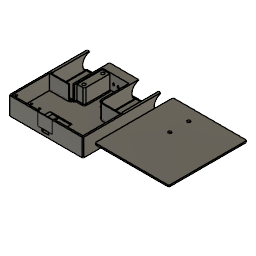
NeoLabs-Rocket-LaunchSystem (Autodesk Fusion 360 design; units mm, degrees)
part number: 2026-06-22-15-23-40-564
Autodesk Fusion 360 part; units mm, degrees
sketch "Sketch1" plane through (0, 0, 0) normal (0, 0, 1) x (1, 0, 0)
  line L0 (-60, -35) -> (39, -35)
  line L1 (39, -35) -> (39, 69.6198)
  line L2 (39, 69.6198) -> (-60, 69.6198)
  line L3 (-60, 69.6198) -> (-60, -35)
  circle A0 centre (-54.5, -30.5) radius 1.35
  circle A1 centre (-34.5, -30.5) radius 1.35
  circle A2 centre (-23.5, -30.5) radius 1.35
  circle A3 centre (-0.5, -30.5) radius 1.35
  dimension "d1" = 99
  dimension "d9" = 2.7
  dimension "d10" = 2.7
  dimension "d11" = 2.7
  dimension "d12" = 2.7
  constraint horizontal L0
  constraint vertical L1
  constraint horizontal L2
  constraint vertical L3
  measures "d1" distance of L0.start L0.end
  measures "d9" diameter of A0
  measures "d10" diameter of A1
  measures "d11" diameter of A2
  measures "d12" diameter of A3
extrude "Extrude1" add sketch "Sketch1" against normal blind 4 makes body 1
extrude "Extrude2" add sketch "Sketch1" along normal blind 6 and the other way blind 4 contours A0 | A1 | A2 | A3 bodies 1
sketch "Sketch2" plane through (0, 0, 0) normal (0, 0, 1) x (-1, 0, 0)
  line L0 (60, -69.6198) -> (60, 35)
  line L1 (60, 35) -> (-39, 35)
  line L2 (-39, 35) -> (-39, -69.6198)
  line L3 (-39, -69.6198) -> (60, -69.6198)
  circle A0 centre (0.5, 30.5) radius 1.35
  circle A1 centre (34.5, 30.5) radius 1.35
  circle A2 centre (54.5, 30.5) radius 1.35
  circle A3 centre (23.5, 30.5) radius 1.35
  line L4 (30.3925, -68.4602) -> (56.3925, -68.4602)
  line L5 (56.3925, -68.4602) -> (56.3925, -20.4602)
  line L6 (56.3925, -20.4602) -> (30.3925, -20.4602)
  line L7 (30.3925, -20.4602) -> (30.3925, -68.4602)
  line L8 (31.8289, -17.2317) -> (57.8727, -17.2317)
  line L9 (57.8727, -17.2317) -> (57.8727, -18.2915)
  line L10 (57.8727, -18.2915) -> (31.8289, -18.2915)
  line L11 (31.8289, -18.2915) -> (31.8289, -17.2317)
  line L12 (57.8615, -18.2915) -> (57.8615, -20.4602)
  line L13 (31.8289, -20.7915) -> (31.8289, -21.7915)
  line L14 (59.9993, -21.7915) -> (59.9993, -16.2915)
  line L15 (57.8615, -17.2317) -> (57.8615, -20.4602)
  line L16 (60, -69.6198) -> (58, -69.6198)
  line L17 (60, -21.7915) -> (60, -69.6198)
  line L18 (60, -21.7915) -> (59.9993, -21.7915)
  line L19 (57.9993, -16.2915) -> (57.9993, 33)
  line L20 (57.9993, 35) -> (59.9993, 35)
  line L21 (59.9993, 35) -> (59.9993, -16.2915)
  line L22 (-39, 35) -> (-37, 35)
  line L23 (-3, -69.6198) -> (-39, -69.6198)
  line L24 (-39, -69.6198) -> (-39, 35)
  line L25 (-3, -69.6198) -> (30.1003, -69.6198)
  line L26 (30.1003, -69.6198) -> (30.1003, -67.6198)
  line L27 (58, -69.6198) -> (56.8045, -69.6198)
  line L28 (56.8045, -69.6198) -> (56.8045, -67.6198)
  line L29 (30.3925, -20.4602) -> (57.8727, -20.4602)
  line L30 (57.8727, -20.4602) -> (57.8727, -18.2915)
  line L31 (57.8727, -18.2915) -> (30.3925, -18.2915)
  line L32 (30.3925, -18.2915) -> (30.3925, -20.4602)
  line L33 (-39, 35) -> (60, 35)
  line L34 (60, 35) -> (60, 33)
  line L35 (-39, 0.9412) -> (-39, 35)
  line L36 (60, 33) -> (59.9993, 33)
  line L37 (57.9993, 33) -> (-3, 33)
  line L38 (28.1003, -58.5213) -> (28.1003, -20.4602)
  line L39 (28.1003, -20.4602) -> (30.1003, -20.4602)
  line L40 (30.1003, -20.4602) -> (30.1003, -67.6198)
  line L41 (57.8727, -20.4602) -> (56.8045, -20.4602)
  line L42 (56.8045, -20.4602) -> (56.8045, -67.6198)
  line L43 (28.1003, -58.5213) -> (17.9963, -58.5213)
  line L44 (57.9993, -16.2915) -> (57.9993, -17.2317)
  line L45 (57.9993, -17.2317) -> (57.8727, -17.2317)
  line L46 (-9.1003, -20.4602) -> (-9.1003, -67.6198)
  line L47 (-9.1003, -69.6198) -> (-9.1003, -67.6198)
  line L48 (-35.8045, -20.4602) -> (-35.8045, -67.6198)
  line L49 (-35.8045, -69.6198) -> (-35.8045, -67.6198)
  line L50 (-36.8615, -17.2317) -> (-36.8615, -20.4602)
  line L51 (-35.3925, -20.4602) -> (-9.3925, -20.4602)
  line L52 (-36.8727, -20.4602) -> (-35.8045, -20.4602)
  line L53 (-9.3925, -20.4602) -> (-36.8727, -20.4602)
  line L54 (-36.8727, -18.2915) -> (-10.8289, -18.2915)
  line L55 (-10.8289, -17.2317) -> (-36.8727, -17.2317)
  line L56 (-36.8727, -18.2915) -> (-9.3925, -18.2915)
  line L57 (-9.3925, -18.2915) -> (-9.3925, -20.4602)
  line L58 (-10.8289, -18.2915) -> (-10.8289, -17.2317)
  line L59 (-7.1003, -20.4602) -> (-9.1003, -20.4602)
  line L60 (-7.1003, -58.5213) -> (-7.1003, -20.4602)
  line L61 (-39, -21.7915) -> (-39, -69.6198)
  line L62 (-39, -69.6198) -> (-37, -69.6198)
  line L63 (-37, -69.6198) -> (-35.8045, -69.6198)
  line L64 (-39, -21.7915) -> (-39, 35)
  line L65 (-37, 35) -> (10.5, 35)
  line L66 (-3, 33) -> (-36.8727, 33)
  line L67 (-36.8727, -17.2317) -> (-36.8727, 33)
  line L68 (-7.1003, -58.5213) -> (3.0037, -58.5213)
  line L69 (3.0037, -58.5213) -> (17.9963, -58.5213)
  dimension "d27" = 26
  dimension "d28" = 48
  dimension "d34" = 2
  dimension "d35" = 2
  dimension "d36" = 2
  constraint horizontal L4
  constraint vertical L5
  constraint horizontal L6
  constraint vertical L7
  constraint horizontal L8
  constraint vertical L9
  constraint horizontal L10
  constraint vertical L11
  constraint coincident L10 L12.start
  constraint perpendicular L10 L12
  constraint vertical L13
  constraint vertical L14
  constraint vertical L15
  constraint horizontal L16
  constraint vertical L17
  constraint coincident L0.start L3.end
  constraint vertical L19
  constraint horizontal L20
  constraint vertical L21
  constraint horizontal L22
  constraint horizontal L23
  constraint vertical L24
  constraint coincident L1.end L2.start
  constraint horizontal L25
  constraint vertical L26
  constraint horizontal L27
  constraint vertical L28
  constraint horizontal L29
  constraint vertical L30
  constraint horizontal L31
  constraint vertical L32
  constraint horizontal L33
  constraint vertical L34
  constraint horizontal L36
  constraint vertical L35
  constraint coincident L0 L34.end
  constraint coincident L21 L36.end
  constraint collinear L36 L37
  constraint vertical L38
  constraint horizontal L39
  constraint vertical L40
  constraint horizontal L41
  constraint vertical L42
  constraint coincident L29 L12.end
  constraint horizontal L43
  constraint perpendicular L8 L44
  constraint perpendicular L15 L45
  constraint coincident L8 L15.start
  constraint midpoint L33 L65.end
  constraint perpendicular L66 L67
  measures "d27" distance of L4.start L4.end
  measures "d28" distance of L4.start L6.end
  measures "d34" distance of L0.start L16.end
  measures "d35" distance of L14.end L19.start
  measures "d36" distance of L1.end L22.end
extrude "Extrude3" add sketch "Sketch2" along normal blind 10 contours L8 L10 L11 L15 L31 | L50 L54 L55 L56 L58 bodies 1
extrude "Extrude5" add sketch "Sketch2" along normal blind 2 contours L6 L10 L12 L15 L29 L31 L32 L41 | L50 L51 L52 L53 L54 L56 L57 bodies 1
extrude "Extrude6" add sketch "Sketch2" along normal blind 20 contours L0 L1 L2 L3 L9 L14 L16 L17 L19 L20 L21 L22 L23 L24 L27 L28 L29 L30 L33 L34 L35 L37 L41 L42 L44 L45 L48 L49 L50 L52 L53 L55 L61 L62 L63 L64 L65 L66 L67 | L3 L23 L25 L26 L38 L39 L40 L43 L46 L47 L59 L60 L68 L69 | L10 L12 L15 L29 L30 L31 L41 | L8 L9 L10 L15 L31 | L8 L10 L11 L15 L31 | L50 L54 L55 L56 L58 | A0 | A1 | A2 | A3 bodies 1
sketch "Sketch4" plane through (-60, 0, 0) normal (-1, 0, 0) x (0, -1, 0)
  line L0 (-69.6198, 20) -> (-69.6198, -4)
  line L1 (-69.6198, -4) -> (35, -4)
  line L2 (35, -4) -> (35, 0)
  line L3 (35, 0) -> (-21.7915, 0)
  line L4 (-21.7915, 0) -> (-21.7915, 20)
  line L5 (-21.7915, 20) -> (-69.6198, 20)
  circle A0 centre (-72, 8) radius 10.4908
extrude "Extrude8" cut sketch "Sketch4" against normal blind 106 contours L0 A0 | L0 A0 bodies 1
sketch "Sketch10" plane through (0, 58.5213, 0) normal (0, -1, 0) x (1, 0, 0)
  line L0 (-28.1003, 0) -> (7.1003, 0)
  line L1 (7.1003, 0) -> (7.1003, 20)
  line L2 (7.1003, 20) -> (-28.1003, 20)
  line L3 (-28.1003, 20) -> (-28.1003, 0)
  line L4 (9, 8.3056) -> (-30, 8.3056)
  line L5 (-10.5, 8.3056) -> (-10.5, 11)
  line L6 (-6.2556, 8.3056) -> (-7.4122, 10.4298)
  line L7 (-7.5876, 10.4301) -> (-8.7556, 8.3056)
  arc A0 (-8.7556, 8.3056) -> (-6.2556, 8.3056) centre (-7.5056, 8.3056) ccw
  arc A1 (-7.4122, 10.4298) -> (-7.5876, 10.4301) centre (-7.5, 10.382) ccw
  line L8 (-13.4124, 10.4301) -> (-12.2444, 8.3056)
  line L9 (-14.7444, 8.3056) -> (-13.5878, 10.4298)
  arc A2 (-13.4124, 10.4301) -> (-13.5878, 10.4298) centre (-13.5, 10.382) ccw
  arc A3 (-14.7444, 8.3056) -> (-12.2444, 8.3056) centre (-13.4944, 8.3056) ccw
  dimension "d92" = 2.5
  dimension "d93" = 0.1
  constraint perpendicular L3 L4
  constraint midpoint L4 L5.start
  constraint perpendicular L4 L5
  constraint coincident L4 A0.centre
  constraint coincident L4 L6.start
  constraint coincident L4 L7.end
  constraint tangent L6 A1
  constraint tangent L7 A1
  constraint symmetric L5 L6.start L9.start
  constraint symmetric L5 L7.end L8.end
  constraint symmetric L5 A0 A3
  constraint symmetric L5 L6.end L9.end
  constraint symmetric L5 L7.start L8.start
  constraint symmetric L5 A1 A2
  measures "d92" diameter of A0
  measures "d93" radius of A1
extrude "Extrude15" cut sketch "Sketch10" against normal blind 10 contours L4 L8 L9 A2 | L4 A3 | L4 A0 | L4 L6 L7 A1 bodies 1
fillet "Fillet2" radius 1 8 edges at (37.4022, 69.6198, 18.2172) (-10.5, 69.6198, 18.2172) (-58.4022, 69.6198, 18.2172) (-10.5, 69.6198, -2.2172) (-30.1003, 61.8033, 10.4663) (-56.8045, 61.8033, 10.4663) (35.8045, 61.8033, 10.4663) (9.1003, 61.8033, 10.4663) on bodies 1
sketch "Sketch5" plane through (0, 0, 0) normal (0, 0, 1) x (-1, 0, 0)
  line L0 (6.8, 32.85) -> (15.8, 32.85)
  line L1 (15.8, 32.85) -> (6.8, 32.85)
  line L2 (6.8, 32.85) -> (6.8, 37.441)
  line L3 (6.8, 37.441) -> (15.8, 37.441)
  line L4 (15.8, 37.441) -> (15.8, 32.85)
  circle A0 centre (54.5, 30.5) radius 1.35
  circle A1 centre (34.5, 30.5) radius 1.35
  circle A2 centre (0.5, 30.5) radius 1.35
  circle A3 centre (23.5, 30.5) radius 1.35
  line L5 (29.1003, -65.2135) -> (57.8045, -65.2135)
  spline S0 degree 3 poles (57.8045, -65.2135) (57.6964, -65.2135) (57.5714, -65.179) (57.3554, -65.0637) (57.235, -64.9522) (57.0463, -64.708) (56.9546, -64.5234) (56.8406, -64.1757) (56.8045, -63.9456) (56.8045, -63.7515) knots 0.358129 0.358129 0.358129 0.358129 0.39055 0.39055 0.431579 0.431579 0.483124 0.483124 0.541351 0.541351 0.541351 0.541351
  line L6 (56.8045, -63.7515) -> (56.8045, -20.4602)
  line L7 (56.8045, -20.4602) -> (30.3925, -20.4602)
  line L8 (30.3925, -20.4602) -> (30.3925, -18.2915)
  line L9 (30.3925, -18.2915) -> (31.8289, -18.2915)
  line L10 (31.8289, -18.2915) -> (31.8289, -17.2317)
  line L11 (31.8289, -17.2317) -> (57.9993, -17.2317)
  line L12 (57.9993, -17.2317) -> (57.9993, 33)
  line L13 (57.9993, 33) -> (-36.8727, 33)
  line L14 (-7.1003, -58.5213) -> (28.1003, -58.5213)
  line L15 (28.1003, -58.5213) -> (28.1003, -20.4602)
  line L16 (28.1003, -20.4602) -> (30.1003, -20.4602)
  line L17 (30.1003, -20.4602) -> (30.1003, -63.7515)
  spline S1 degree 3 poles (30.1003, -63.7515) (30.1003, -63.9456) (30.0641, -64.1757) (29.9501, -64.5234) (29.8585, -64.708) (29.6697, -64.9522) (29.5493, -65.0637) (29.3333, -65.179) (29.2083, -65.2135) (29.1003, -65.2135) knots 0.174906 0.174906 0.174906 0.174906 0.233133 0.233133 0.284679 0.284679 0.325708 0.325708 0.358129 0.358129 0.358129 0.358129
  line L18 (-36.8727, 33) -> (-36.8727, -17.2317)
  line L19 (-36.8727, -17.2317) -> (-10.8289, -17.2317)
  line L20 (-10.8289, -17.2317) -> (-10.8289, -18.2915)
  line L21 (-10.8289, -18.2915) -> (-9.3925, -18.2915)
  line L22 (-9.3925, -18.2915) -> (-9.3925, -20.4602)
  line L23 (-9.3925, -20.4602) -> (-35.8045, -20.4602)
  line L24 (-35.8045, -20.4602) -> (-35.8045, -63.7515)
  line L25 (-9.1003, -63.7515) -> (-9.1003, -20.4602)
  line L26 (-9.1003, -20.4602) -> (-7.1003, -20.4602)
  line L27 (-7.1003, -20.4602) -> (-7.1003, -58.5213)
  spline S2 degree 3 poles (-35.8045, -63.7515) (-35.8045, -63.9456) (-35.8406, -64.1757) (-35.9546, -64.5234) (-36.0463, -64.708) (-36.235, -64.9522) (-36.3554, -65.0637) (-36.5714, -65.179) (-36.6964, -65.2135) (-36.8045, -65.2135) knots 0.174906 0.174906 0.174906 0.174906 0.233133 0.233133 0.284679 0.284679 0.325708 0.325708 0.358129 0.358129 0.358129 0.358129
  line L28 (-36.8045, -65.2135) -> (-8.1003, -65.2135)
  spline S3 degree 3 poles (-8.1003, -65.2135) (-8.2083, -65.2135) (-8.3333, -65.179) (-8.5493, -65.0637) (-8.6697, -64.9522) (-8.8585, -64.708) (-8.9501, -64.5234) (-9.0641, -64.1757) (-9.1003, -63.9456) (-9.1003, -63.7515) knots 0.358129 0.358129 0.358129 0.358129 0.39055 0.39055 0.431579 0.431579 0.483124 0.483124 0.541351 0.541351 0.541351 0.541351
  dimension "d60" = 9
  constraint horizontal L1
  constraint vertical L2
  constraint horizontal L3
  constraint vertical L4
  measures "d60" distance of L0.start L0.end
extrude "Extrude9" cut sketch "Sketch5" along normal blind 3.2 contours L2 L3 L4 L13 bodies 1
sketch "Sketch6" plane through (0, 0, 20) normal (0, 0, 1) x (-1, 0, 0)
  line L0 (56.8045, -69.6198) -> (60, -69.6198)
  line L1 (60, -69.6198) -> (60, -21.7915)
  line L2 (60, -21.7915) -> (59.9993, -21.7915)
  line L3 (59.9993, -21.7915) -> (59.9993, 35)
  line L4 (59.9993, 35) -> (-39, 35)
  line L5 (-39, 35) -> (-39, -69.6198)
  line L6 (21.6224, 33) -> (2.3035, 33)
  line L7 (2.3035, 33) -> (2.3035, 34.4706)
  line L8 (2.3035, 34.4706) -> (21.6224, 34.4706)
  line L9 (21.6224, 34.4706) -> (21.6224, 33)
  line L10 (-36.8727, 33) -> (57.9993, 33)
  line L11 (57.9993, 33) -> (57.9993, -17.2317)
  line L12 (57.9993, -17.2317) -> (31.8289, -17.2317)
  line L13 (31.8289, -17.2317) -> (31.8289, -18.2915)
  line L14 (31.8289, -18.2915) -> (57.8615, -18.2915)
  line L15 (57.8615, -18.2915) -> (57.8615, -20.4602)
  line L16 (57.8615, -20.4602) -> (56.8045, -20.4602)
  line L17 (56.8045, -20.4602) -> (56.8045, -69.6198)
  line L18 (-39, -69.6198) -> (-35.8045, -69.6198)
  line L19 (-36.8615, -18.2915) -> (-10.8289, -18.2915)
  line L20 (-10.8289, -18.2915) -> (-10.8289, -17.2317)
  line L21 (-10.8289, -17.2317) -> (-36.8727, -17.2317)
  line L22 (-36.8727, -17.2317) -> (-36.8727, 33)
  line L23 (-35.8045, -69.6198) -> (-35.8045, -20.4602)
  line L24 (-35.8045, -20.4602) -> (-36.8615, -20.4602)
  line L25 (-36.8615, -20.4602) -> (-36.8615, -18.2915)
  constraint horizontal L6
  constraint vertical L7
  constraint horizontal L8
  constraint vertical L9
extrude "Extrude10" cut sketch "Sketch6" against normal blind 17 contours L6 L7 L8 L9 L10 bodies 1
fillet "Fillet3" radius 0.5 4 edges at (-1.7586, -30.0118, 0) (-24.7586, -30.0118, 0) (-35.7586, -30.0118, 0) (-55.7586, -30.0118, 0) on bodies 1
sketch "Sketch7" plane through (0, 0, 0) normal (0, 0, 1) x (-1, 0, 0)
  circle A0 centre (34.5, 30.5) radius 1.85
  circle A1 centre (0.5, 30.5) radius 1.85
  line L0 (29.1003, -65.2135) -> (57.8045, -65.2135)
  spline S0 degree 3 poles (57.8045, -65.2135) (57.6964, -65.2135) (57.5714, -65.179) (57.3554, -65.0637) (57.235, -64.9522) (57.0463, -64.708) (56.9546, -64.5234) (56.8406, -64.1757) (56.8045, -63.9456) (56.8045, -63.7515) knots 0.358129 0.358129 0.358129 0.358129 0.39055 0.39055 0.431579 0.431579 0.483124 0.483124 0.541351 0.541351 0.541351 0.541351
  line L1 (56.8045, -63.7515) -> (56.8045, -20.4602)
  line L2 (56.8045, -20.4602) -> (30.3925, -20.4602)
  line L3 (30.3925, -20.4602) -> (30.3925, -18.2915)
  line L4 (30.3925, -18.2915) -> (31.8289, -18.2915)
  line L5 (31.8289, -18.2915) -> (31.8289, -17.2317)
  line L6 (31.8289, -17.2317) -> (57.9993, -17.2317)
  line L7 (57.9993, -17.2317) -> (57.9993, 33)
  line L8 (57.9993, 33) -> (15.8, 33)
  line L9 (15.8, 33) -> (15.8, 35)
  line L10 (15.8, 35) -> (6.8, 35)
  line L11 (6.8, 35) -> (6.8, 33)
  line L12 (6.8, 33) -> (-36.8727, 33)
  line L13 (-7.1003, -58.5213) -> (28.1003, -58.5213)
  line L14 (28.1003, -58.5213) -> (28.1003, -20.4602)
  line L15 (28.1003, -20.4602) -> (30.1003, -20.4602)
  line L16 (30.1003, -20.4602) -> (30.1003, -63.7515)
  spline S1 degree 3 poles (30.1003, -63.7515) (30.1003, -63.9456) (30.0641, -64.1757) (29.9501, -64.5234) (29.8585, -64.708) (29.6697, -64.9522) (29.5493, -65.0637) (29.3333, -65.179) (29.2083, -65.2135) (29.1003, -65.2135) knots 0.174906 0.174906 0.174906 0.174906 0.233133 0.233133 0.284679 0.284679 0.325708 0.325708 0.358129 0.358129 0.358129 0.358129
  circle A2 centre (23.5, 30.5) radius 1.85
  circle A3 centre (54.5, 30.5) radius 1.85
  circle A4 centre (22.12, -52.8277) radius 2.05
  line L17 (27, -57) -> (17, -57)
  line L18 (17, -57) -> (17, -23)
  line L19 (17, -23) -> (27, -23)
  line L20 (27, -23) -> (27, -57)
  circle A5 centre (22.0931, -27.4434) radius 2.05
  line L21 (-36.8727, 33) -> (-36.8727, -17.2317)
  line L22 (-36.8727, -17.2317) -> (-10.8289, -17.2317)
  line L23 (-10.8289, -17.2317) -> (-10.8289, -18.2915)
  line L24 (-10.8289, -18.2915) -> (-9.3925, -18.2915)
  line L25 (-9.3925, -18.2915) -> (-9.3925, -20.4602)
  line L26 (-9.3925, -20.4602) -> (-35.8045, -20.4602)
  line L27 (-35.8045, -20.4602) -> (-35.8045, -63.7515)
  line L28 (-9.1003, -63.7515) -> (-9.1003, -20.4602)
  line L29 (-9.1003, -20.4602) -> (-7.1003, -20.4602)
  line L30 (-7.1003, -20.4602) -> (-7.1003, -58.5213)
  spline S2 degree 3 poles (-35.8045, -63.7515) (-35.8045, -63.9456) (-35.8406, -64.1757) (-35.9546, -64.5234) (-36.0463, -64.708) (-36.235, -64.9522) (-36.3554, -65.0637) (-36.5714, -65.179) (-36.6964, -65.2135) (-36.8045, -65.2135) knots 0.174906 0.174906 0.174906 0.174906 0.233133 0.233133 0.284679 0.284679 0.325708 0.325708 0.358129 0.358129 0.358129 0.358129
  line L31 (-36.8045, -65.2135) -> (-8.1003, -65.2135)
  spline S3 degree 3 poles (-8.1003, -65.2135) (-8.2083, -65.2135) (-8.3333, -65.179) (-8.5493, -65.0637) (-8.6697, -64.9522) (-8.8585, -64.708) (-8.9501, -64.5234) (-9.0641, -64.1757) (-9.1003, -63.9456) (-9.1003, -63.7515) knots 0.358129 0.358129 0.358129 0.358129 0.39055 0.39055 0.431579 0.431579 0.483124 0.483124 0.541351 0.541351 0.541351 0.541351
  dimension "d67" = 4.1
  dimension "d70" = 4.1
  constraint horizontal L17
  constraint vertical L18
  constraint horizontal L19
  constraint vertical L20
  measures "d67" diameter of A4
  measures "d70" diameter of A5
extrude "Extrude11" add sketch "Sketch7" along normal blind 20 contours L17 L18 L19 L20 bodies 1
extrude "Extrude12" add sketch "Sketch7" along normal blind 14 contours A4 | A5 bodies 1
fillet "Fillet4" radius 2 1 edges at (-17, 23, 10) on bodies 1
fillet "Fillet5" radius 0.5 8 edges at (-30.1003, 20.4602, 10) (-31.8289, 18.2915, 11) (-31.8289, 17.2317, 10) (-28.1003, 20.4602, 10) (7.1003, 20.4602, 10) (9.1003, 20.4602, 10) (10.8289, 18.2915, 11) (10.8289, 17.2317, 10) on bodies 1
fillet "Fillet6" radius 0.25 2 edges at (-30.3925, 18.2915, 1) (9.3925, 18.2915, 1) on bodies 1
fillet "Fillet7" radius 1 3 edges at (-17, 41, 0) (-17.5858, 23.5858, 0) (-23, 23, 0) on bodies 1
fillet "Fillet8" radius 0.5 16 edges at (-57.0463, 64.6852, 0) (-56.8045, 42.1058, 0) (-28.1003, 39.7407, 0) (-28.2467, 20.6066, 0) (-29.1003, 20.4602, 0) (-29.9538, 20.6066, 0) (-30.1003, 42.3558, 0) (-29.8584, 64.6852, 0) (8.8584, 64.6852, 0) (9.1003, 42.3558, 0) (8.9538, 20.6066, 0) (8.1003, 20.4602, 0) (7.2467, 20.6066, 0) (7.1003, 39.7407, 0) (35.8045, 42.1058, 0) (36.0463, 64.6852, 0) on bodies 1
chamfer "Chamfer1" distance 1 angle 45 13 edges at (39, -35, 8) (39, 69.6198, -3.4912) (39, 69.4242, -2.3883) (39, 61.5092, 8) (39, 69.4242, 18.3883) (39, 69.6198, 19.4912) (-59.9993, -35, 10) (-60, -35, -2) (-60, 69.6198, 19.4912) (-60, 69.4242, 18.3883) (-60, 61.5092, 8) (-60, 69.4242, -2.3883) (-60, 69.6198, -3.4912) on bodies 1
sketch "Sketch9" plane through (0, 0, 0) normal (0, 0, 1) x (-1, 0, 0)
  line L0 (27, -22) -> (27, -57)
  line L1 (27, -57) -> (16, -57)
  line L2 (16, -57) -> (16, -25)
  arc A0 (19, -22) -> (16, -25) centre (19, -25) ccw
  line L3 (19, -22) -> (27, -22)
  circle A1 centre (54.5, 30.5) radius 1.85
  circle A2 centre (23.5, 30.5) radius 1.85
  line L4 (27.6003, -58.5213) -> (27.6003, -20.9602)
  arc A3 (28.6003, -19.9602) -> (27.6003, -20.9602) centre (28.6003, -20.9602) ccw
  line L5 (28.6003, -19.9602) -> (29.6003, -19.9602)
  arc A4 (30.3925, -20.3499) -> (29.6003, -19.9602) centre (29.6003, -20.9602) ccw
  line L6 (30.3925, -20.3499) -> (30.3925, -18.5415)
  arc A5 (30.6425, -18.2915) -> (30.3925, -18.5415) centre (30.6425, -18.5415) ccw
  line L7 (30.6425, -18.2915) -> (31.8289, -18.2915)
  line L8 (31.8289, -18.2915) -> (31.8289, -17.7317)
  arc A6 (32.3289, -17.2317) -> (31.8289, -17.7317) centre (32.3289, -17.7317) ccw
  line L9 (32.3289, -17.2317) -> (57.9993, -17.2317)
  line L10 (57.9993, -17.2317) -> (57.9993, 33)
  line L11 (57.9993, 33) -> (15.8, 33)
  line L12 (15.8, 33) -> (15.8, 35)
  line L13 (15.8, 35) -> (6.8, 35)
  line L14 (6.8, 35) -> (6.8, 33)
  line L15 (6.8, 33) -> (-36.8727, 33)
  line L16 (-6.6003, -58.5213) -> (27.6003, -58.5213)
  circle A7 centre (0.5, 30.5) radius 1.85
  circle A8 centre (34.5, 30.5) radius 1.85
  line L17 (10.6673, -61.4434) -> (10.6673, -26.1703) construction
  line L18 (10.6673, -26.1703) -> (0.8534, -26.1703) construction
  line L19 (0.8534, -26.1703) -> (0.8534, -61.4434) construction
  line L20 (0.8534, -61.4434) -> (10.6673, -61.4434) construction
  line L21 (-36.8727, 33) -> (-36.8727, -17.2317)
  line L22 (-36.8727, -17.2317) -> (-11.3289, -17.2317)
  line L23 (-10.8289, -17.7317) -> (-10.8289, -18.2915)
  line L24 (-10.8289, -18.2915) -> (-9.6425, -18.2915)
  line L25 (-9.3925, -18.5415) -> (-9.3925, -20.3499)
  arc A9 (-10.8289, -17.7317) -> (-11.3289, -17.2317) centre (-11.3289, -17.7317) ccw
  arc A10 (-9.3925, -18.5415) -> (-9.6425, -18.2915) centre (-9.6425, -18.5415) ccw
  line L26 (-6.6003, -20.9602) -> (-6.6003, -58.5213)
  arc A11 (-8.6003, -19.9602) -> (-9.3925, -20.3499) centre (-8.6003, -20.9602) ccw
  line L27 (-8.6003, -19.9602) -> (-7.6003, -19.9602)
  arc A12 (-6.6003, -20.9602) -> (-7.6003, -19.9602) centre (-7.6003, -20.9602) ccw
  dimension "d88" = 5
  text T0 "Made by Neo" font "Arial" height 5 align centre middle in box 35.273 x 9.8139 at (10.6673, -61.4434) x (0, 1) y (-1, 0) spacing 1 kerned
extrude "Extrude14" cut sketch "Sketch9" against normal blind 1 text T0 bodies 1
sketch "Sketch11" plane through (0, 0, 0) normal (0, 0, 1) x (-1, 0, 0)
  circle A0 centre (34.5, 30.5) radius 1.85
  circle A1 centre (0.5, 30.5) radius 1.85
  line L0 (27.6003, -58.5213) -> (27.6003, -20.9602)
  arc A2 (28.6003, -19.9602) -> (27.6003, -20.9602) centre (28.6003, -20.9602) ccw
  line L1 (28.6003, -19.9602) -> (29.6003, -19.9602)
  arc A3 (30.3925, -20.3499) -> (29.6003, -19.9602) centre (29.6003, -20.9602) ccw
  line L2 (30.3925, -20.3499) -> (30.3925, -18.5415)
  arc A4 (30.6425, -18.2915) -> (30.3925, -18.5415) centre (30.6425, -18.5415) ccw
  line L3 (30.6425, -18.2915) -> (31.8289, -18.2915)
  line L4 (31.8289, -18.2915) -> (31.8289, -17.7317)
  arc A5 (32.3289, -17.2317) -> (31.8289, -17.7317) centre (32.3289, -17.7317) ccw
  line L5 (32.3289, -17.2317) -> (57.9993, -17.2317)
  line L6 (57.9993, -17.2317) -> (57.9993, 33)
  line L7 (57.9993, 33) -> (15.8, 33)
  line L8 (15.8, 33) -> (15.8, 35)
  line L9 (15.8, 35) -> (6.8, 35)
  line L10 (6.8, 35) -> (6.8, 33)
  line L11 (6.8, 33) -> (-36.8727, 33)
  line L12 (-36.8727, 33) -> (-36.8727, -17.2317)
  line L13 (-36.8727, -17.2317) -> (-11.3289, -17.2317)
  line L14 (-10.8289, -17.7317) -> (-10.8289, -18.2915)
  line L15 (-10.8289, -18.2915) -> (-9.6425, -18.2915)
  line L16 (-9.3925, -18.5415) -> (-9.3925, -20.3499)
  line L17 (-6.6003, -58.5213) -> (27.6003, -58.5213)
  circle A6 centre (23.5, 30.5) radius 1.85
  circle A7 centre (54.5, 30.5) radius 1.85
  line L18 (27, -22) -> (27, -57)
  line L19 (27, -57) -> (16, -57)
  line L20 (16, -57) -> (16, -25)
  arc A8 (19, -22) -> (16, -25) centre (19, -25) ccw
  line L21 (19, -22) -> (27, -22)
  line L22 (0.1021, -56.2744) -> (4.3585, -56.2744)
  line L23 (4.3585, -56.2744) -> (4.3585, -56.9122)
  line L24 (4.3585, -56.9122) -> (-0.6415, -56.9122)
  line L25 (-0.6415, -56.9122) -> (-0.6415, -55.9163)
  line L26 (-0.6415, -55.9163) -> (2.8988, -54.7328)
  spline S0 degree 3 poles (2.8988, -54.7328) (3.0427, -54.6852) (3.2889, -54.6038) (3.5362, -54.5263) (3.6389, -54.4941) knots 0 0 0 0 0.045488 0.077767 0.077767 0.077767 0.077767
  spline S1 degree 3 poles (3.6389, -54.4941) (3.5265, -54.458) (3.2585, -54.3719) (2.9921, -54.2809) (2.8374, -54.2281) knots 0 0 0 0 0.035404 0.084451 0.084451 0.084451 0.084451
  line L27 (2.8374, -54.2281) -> (-0.6415, -53.0309)
  line L28 (-0.6415, -53.0309) -> (-0.6415, -52.1408)
  line L29 (-0.6415, -52.1408) -> (4.3585, -52.1408)
  line L30 (4.3585, -52.1408) -> (4.3585, -52.7785)
  line L31 (4.3585, -52.7785) -> (0.1737, -52.7785)
  line L32 (0.1737, -52.7785) -> (4.3585, -54.2315)
  line L33 (4.3585, -54.2315) -> (4.3585, -54.8283)
  line L34 (4.3585, -54.8283) -> (0.1021, -56.2744)
  line L35 (-0.6415, -44.3474) -> (4.3585, -44.3474)
  line L36 (4.3585, -44.3474) -> (4.3585, -44.917)
  line L37 (4.3585, -44.917) -> (3.9015, -44.917)
  spline S2 degree 3 poles (3.9015, -44.917) (4.0587, -45.0468) (4.3773, -45.3099) (4.4192, -45.7214) (4.4404, -45.93) knots 0 0 0 0 0.058684 0.118957 0.118957 0.118957 0.118957
  spline S3 degree 3 poles (4.4404, -45.93) (4.4304, -46.0715) (4.4104, -46.3548) (4.2713, -46.6024) (4.2017, -46.7264) knots 0 0 0 0 0.041993 0.084065 0.084065 0.084065 0.084065
  spline S4 degree 3 poles (4.2017, -46.7264) (4.1127, -46.8413) (3.9307, -47.0764) (3.6687, -47.2172) (3.5349, -47.2891) knots 0 0 0 0 0.043095 0.088123 0.088123 0.088123 0.088123
  spline S5 degree 3 poles (3.5349, -47.2891) (3.3833, -47.3473) (3.0667, -47.4687) (2.7276, -47.4818) (2.5509, -47.4886) knots 0 0 0 0 0.048374 0.101007 0.101007 0.101007 0.101007
  spline S6 degree 3 poles (2.5509, -47.4886) (2.3769, -47.4821) (2.04, -47.4696) (1.7211, -47.3606) (1.5669, -47.3079) knots 0 0 0 0 0.051911 0.100523 0.100523 0.100523 0.100523
  spline S7 degree 3 poles (1.5669, -47.3079) (1.4294, -47.2418) (1.1617, -47.1131) (0.9789, -46.8793) (0.8899, -46.7656) knots 0 0 0 0 0.045081 0.087788 0.087788 0.087788 0.087788
  spline S8 degree 3 poles (0.8899, -46.7656) (0.8213, -46.6408) (0.6827, -46.389) (0.664, -46.1021) (0.6546, -45.9573) knots 0 0 0 0 0.042157 0.08511 0.08511 0.08511 0.08511
  spline S9 degree 3 poles (0.6546, -45.9573) (0.6596, -45.8525) (0.6693, -45.6494) (0.7524, -45.4639) (0.7927, -45.374) knots 0 0 0 0 0.031144 0.060409 0.060409 0.060409 0.060409
  spline S10 degree 3 poles (0.7927, -45.374) (0.8416, -45.2932) (0.938, -45.134) (1.0818, -45.016) (1.1525, -44.9579) knots 0 0 0 0 0.028121 0.055368 0.055368 0.055368 0.055368
  line L38 (1.1525, -44.9579) -> (-0.6415, -44.9579)
  line L39 (-0.6415, -44.9579) -> (-0.6415, -44.3474)
  spline S11 degree 3 poles (12.2439, -39.5828) (12.2264, -39.8214) (12.1926, -40.2833) (11.8984, -40.6399) (11.7562, -40.8123) knots 0 0 0 0 0.06984 0.135217 0.135217 0.135217 0.135217
  spline S12 degree 3 poles (11.7562, -40.8123) (11.5646, -40.9488) (11.1462, -41.247) (10.6306, -41.2692) (10.351, -41.2813) knots 0 0 0 0 0.069132 0.150979 0.150979 0.150979 0.150979
  spline S13 degree 3 poles (10.351, -41.2813) (10.0462, -41.2673) (9.4854, -41.2415) (9.0564, -40.8847) (8.8606, -40.7219) knots 0 0 0 0 0.088678 0.163104 0.163104 0.163104 0.163104
  spline S14 degree 3 poles (8.8606, -40.7219) (8.7432, -40.5551) (8.5028, -40.2135) (8.4733, -39.7963) (8.4581, -39.5828) knots 0 0 0 0 0.059989 0.122873 0.122873 0.122873 0.122873
  spline S15 degree 3 poles (8.4581, -39.5828) (8.4763, -39.3473) (8.5118, -38.8883) (8.8048, -38.5342) (8.9476, -38.3618) knots 0 0 0 0 0.068966 0.13445 0.13445 0.13445 0.13445
  spline S16 degree 3 poles (8.9476, -38.3618) (9.1347, -38.2236) (9.5352, -37.928) (10.0341, -37.9017) (10.2999, -37.8877) knots 0 0 0 0 0.068269 0.146129 0.146129 0.146129 0.146129
  spline S17 degree 3 poles (10.2999, -37.8877) (10.5108, -37.8918) (10.8902, -37.8991) (11.2431, -38.0365) (11.3998, -38.0974) knots 0 0 0 0 0.062677 0.112749 0.112749 0.112749 0.112749
  spline S18 degree 3 poles (11.3998, -38.0974) (11.5261, -38.1755) (11.7794, -38.3322) (11.9411, -38.5824) (12.0223, -38.7079) knots 0 0 0 0 0.043935 0.088163 0.088163 0.088163 0.088163
  spline S19 degree 3 poles (12.0223, -38.7079) (12.0869, -38.8453) (12.2174, -39.1225) (12.235, -39.4284) (12.2439, -39.5828) knots 0 0 0 0 0.045086 0.090996 0.090996 0.090996 0.090996
  spline S20 degree 3 poles (5.687, -32.799) (5.7283, -32.8746) (5.814, -33.0318) (5.8236, -33.2109) (5.8285, -33.3038) knots 0 0 0 0 0.025506 0.05302 0.05302 0.05302 0.05302
  spline S21 degree 3 poles (5.8285, -33.3038) (5.8246, -33.3667) (5.8163, -33.5017) (5.7754, -33.6306) (5.7535, -33.6994) knots 0 0 0 0 0.018852 0.040405 0.040405 0.040405 0.040405
  line L40 (5.7535, -33.6994) -> (5.1771, -33.7676)
  spline S22 degree 3 poles (5.1771, -33.7676) (5.193, -33.7052) (5.2223, -33.5897) (5.2287, -33.4709) (5.2317, -33.4163) knots 0 0 0 0 0.019283 0.035626 0.035626 0.035626 0.035626
  spline S23 degree 3 poles (5.2317, -33.4163) (5.2301, -33.354) (5.2273, -33.2405) (5.1833, -33.136) (5.1635, -33.0889) knots 0 0 0 0 0.018496 0.033707 0.033707 0.033707 0.033707
  spline S24 degree 3 poles (5.1635, -33.0889) (5.1382, -33.0497) (5.0874, -32.9705) (5.011, -32.9155) (4.9725, -32.8877) knots 0 0 0 0 0.013848 0.027964 0.027964 0.027964 0.027964
  spline S25 degree 3 poles (4.9725, -32.8877) (4.9194, -32.8616) (4.7714, -32.7888) (4.6154, -32.7348) (4.5154, -32.7001) knots 0 0 0 0 0.017736 0.049441 0.049441 0.049441 0.049441
  spline S26 degree 3 poles (4.5154, -32.7001) (4.4944, -32.6928) (4.4441, -32.6753) (4.3943, -32.6565) (4.3654, -32.6455) knots 0 0 0 0 0.006688 0.015969 0.015969 0.015969 0.015969
  line L41 (4.3654, -32.6455) -> (0.7364, -34.02)
  line L42 (0.7364, -34.02) -> (0.7364, -33.3584)
  line L43 (0.7364, -33.3584) -> (2.834, -32.6046)
  spline S27 degree 3 poles (2.834, -32.6046) (2.9699, -32.5567) (3.2465, -32.4592) (3.5292, -32.3815) (3.673, -32.342) knots 0 0 0 0 0.043223 0.08794 0.08794 0.08794 0.08794
  spline S28 degree 3 poles (3.673, -32.342) (3.5332, -32.3051) (3.2548, -32.2318) (2.9829, -32.1369) (2.8476, -32.0896) knots 0 0 0 0 0.04336 0.08634 0.08634 0.08634 0.08634
  line L44 (2.8476, -32.0896) -> (0.7364, -31.3154)
  line L45 (0.7364, -31.3154) -> (0.7364, -30.7015)
  line L46 (0.7364, -30.7015) -> (4.4199, -32.0794)
  spline S29 degree 3 poles (4.4199, -32.0794) (4.5892, -32.1419) (4.8682, -32.245) (5.1364, -32.3734) (5.2419, -32.4238) knots 0 0 0 0 0.054105 0.089163 0.089163 0.089163 0.089163
  spline S30 degree 3 poles (5.2419, -32.4238) (5.3341, -32.4772) (5.5049, -32.576) (5.6296, -32.7287) (5.687, -32.799) knots 0 0 0 0 0.03163 0.058639 0.058639 0.058639 0.058639
  spline S31 degree 3 poles (11.7392, -43.4129) (11.7328, -43.306) (11.7206, -43.0991) (11.6135, -42.922) (11.5618, -42.8365) knots 0 0 0 0 0.031605 0.06112 0.06112 0.06112 0.06112
  spline S32 degree 3 poles (11.5618, -42.8365) (11.489, -42.7594) (11.3297, -42.5906) (11.1132, -42.5046) (10.9957, -42.4579) knots 0 0 0 0 0.031433 0.068842 0.068842 0.068842 0.068842
  line L47 (10.9957, -42.4579) -> (11.0741, -41.8236)
  spline S33 degree 3 poles (11.0741, -41.8236) (11.2472, -41.8818) (11.5821, -41.9946) (11.8214, -42.2541) (11.937, -42.3795) knots 0 0 0 0 0.053808 0.104129 0.104129 0.104129 0.104129
  spline S34 degree 3 poles (11.937, -42.3795) (12.0264, -42.5296) (12.2163, -42.8484) (12.2344, -43.2199) (12.2439, -43.4163) knots 0 0 0 0 0.051631 0.10961 0.10961 0.10961 0.10961
  spline S35 degree 3 poles (12.2439, -43.4163) (12.2276, -43.6635) (12.1962, -44.1363) (11.8972, -44.5021) (11.7545, -44.6766) knots 0 0 0 0 0.072283 0.138227 0.138227 0.138227 0.138227
  spline S36 degree 3 poles (11.7545, -44.6766) (11.5654, -44.8122) (11.1567, -45.1051) (10.6526, -45.1292) (10.3817, -45.1421) knots 0 0 0 0 0.068378 0.147723 0.147723 0.147723 0.147723
  spline S37 degree 3 poles (10.3817, -45.1421) (10.1019, -45.1293) (9.5826, -45.1056) (9.1585, -44.8085) (8.9629, -44.6714) knots 0 0 0 0 0.082022 0.152248 0.152248 0.152248 0.152248
  spline S38 degree 3 poles (8.9629, -44.6714) (8.8157, -44.5001) (8.5141, -44.149) (8.4771, -43.6869) (8.4581, -43.4504) knots 0 0 0 0 0.065997 0.135199 0.135199 0.135199 0.135199
  spline S39 degree 3 poles (8.4581, -43.4504) (8.477, -43.221) (8.5139, -42.7714) (8.8085, -42.4305) (8.9527, -42.2635) knots 0 0 0 0 0.067144 0.131583 0.131583 0.131583 0.131583
  spline S40 degree 3 poles (8.9527, -42.2635) (9.1445, -42.1295) (9.5605, -41.8386) (10.0697, -41.8155) (10.3442, -41.8031) knots 0 0 0 0 0.068809 0.149275 0.149275 0.149275 0.149275
  spline S41 degree 3 poles (10.3442, -41.8031) (10.367, -41.8033) (10.4215, -41.8038) (10.4761, -41.8055) (10.5079, -41.8065) knots 0 0 0 0 0.006822 0.016375 0.016375 0.016375 0.016375
  line L48 (10.5079, -41.8065) -> (10.5079, -44.5077)
  spline S42 degree 3 poles (10.5079, -44.5077) (10.6898, -44.49) (11.0254, -44.4573) (11.2974, -44.2603) (11.422, -44.1701) knots 0 0 0 0 0.053662 0.09901 0.09901 0.09901 0.09901
  spline S43 degree 3 poles (11.422, -44.1701) (11.5145, -44.062) (11.7012, -43.8437) (11.7264, -43.5574) (11.7392, -43.4129) knots 0 0 0 0 0.041583 0.083942 0.083942 0.083942 0.083942
  line L49 (8.233, -49.2758) -> (12.1621, -49.2758)
  line L50 (12.1621, -49.2758) -> (12.1621, -49.9102)
  line L51 (12.1621, -49.9102) -> (7.1621, -49.9102)
  line L52 (7.1621, -49.9102) -> (7.1621, -49.2315)
  line L53 (7.1621, -49.2315) -> (11.0877, -46.6053)
  line L54 (11.0877, -46.6053) -> (7.1621, -46.6053)
  line L55 (7.1621, -46.6053) -> (7.1621, -45.9709)
  line L56 (7.1621, -45.9709) -> (12.1621, -45.9709)
  line L57 (12.1621, -45.9709) -> (12.1621, -46.6496)
  line L58 (12.1621, -46.6496) -> (8.233, -49.2758)
  spline S44 degree 3 poles (4.4404, -35.9845) (4.4178, -36.187) (4.3725, -36.5931) (4.0611, -36.8579) (3.9049, -36.9907) knots 0 0 0 0 0.058759 0.117889 0.117889 0.117889 0.117889
  line L59 (3.9049, -36.9907) -> (4.3585, -36.9907)
  line L60 (4.3585, -36.9907) -> (4.3585, -37.5603)
  line L61 (4.3585, -37.5603) -> (-0.6415, -37.5603)
  line L62 (-0.6415, -37.5603) -> (-0.6415, -36.9463)
  line L63 (-0.6415, -36.9463) -> (1.1423, -36.9463)
  spline S45 degree 3 poles (1.1423, -36.9463) (1.0001, -36.8088) (0.7182, -36.5362) (0.6757, -36.1467) (0.6546, -35.9538) knots 0 0 0 0 0.057414 0.113746 0.113746 0.113746 0.113746
  spline S46 degree 3 poles (0.6546, -35.9538) (0.6601, -35.8442) (0.671, -35.626) (0.75, -35.4224) (0.7893, -35.3212) knots 0 0 0 0 0.032703 0.065059 0.065059 0.065059 0.065059
  spline S47 degree 3 poles (0.7893, -35.3212) (0.8382, -35.2266) (0.9347, -35.0398) (1.0909, -34.8993) (1.1679, -34.83) knots 0 0 0 0 0.031659 0.062469 0.062469 0.062469 0.062469
  spline S48 degree 3 poles (1.1679, -34.83) (1.2554, -34.7687) (1.4375, -34.641) (1.6473, -34.5667) (1.7562, -34.5282) knots 0 0 0 0 0.03192 0.066398 0.066398 0.066398 0.066398
  spline S49 degree 3 poles (1.7562, -34.5282) (1.8743, -34.4964) (2.1156, -34.4314) (2.3654, -34.4232) (2.4929, -34.4191) knots 0 0 0 0 0.036569 0.074696 0.074696 0.074696 0.074696
  spline S50 degree 3 poles (2.4929, -34.4191) (2.777, -34.4309) (3.3012, -34.4528) (3.734, -34.7455) (3.9322, -34.8795) knots 0 0 0 0 0.083336 0.153774 0.153774 0.153774 0.153774
  spline S51 degree 3 poles (3.9322, -34.8795) (4.0804, -35.0387) (4.3717, -35.3516) (4.4178, -35.776) (4.4404, -35.9845) knots 0 0 0 0 0.063387 0.124577 0.124577 0.124577 0.124577
  spline S52 degree 3 poles (3.9356, -41.8577) (3.9293, -41.7507) (3.9171, -41.5439) (3.81, -41.3668) (3.7583, -41.2813) knots 0 0 0 0 0.031605 0.06112 0.06112 0.06112 0.06112
  spline S53 degree 3 poles (3.7583, -41.2813) (3.6855, -41.2042) (3.5261, -41.0353) (3.3097, -40.9494) (3.1921, -40.9027) knots 0 0 0 0 0.031433 0.068842 0.068842 0.068842 0.068842
  line L64 (3.1921, -40.9027) -> (3.2705, -40.2683)
  spline S54 degree 3 poles (3.2705, -40.2683) (3.4436, -40.3266) (3.7786, -40.4394) (4.0178, -40.6989) (4.1334, -40.8242) knots 0 0 0 0 0.053808 0.104129 0.104129 0.104129 0.104129
  spline S55 degree 3 poles (4.1334, -40.8242) (4.2229, -40.9744) (4.4128, -41.2932) (4.4308, -41.6646) (4.4404, -41.8611) knots 0 0 0 0 0.051631 0.10961 0.10961 0.10961 0.10961
  spline S56 degree 3 poles (4.4404, -41.8611) (4.424, -42.1083) (4.3927, -42.5811) (4.0936, -42.9468) (3.951, -43.1213) knots 0 0 0 0 0.072283 0.138227 0.138227 0.138227 0.138227
  spline S57 degree 3 poles (3.951, -43.1213) (3.7618, -43.2569) (3.3532, -43.5498) (2.849, -43.5739) (2.5782, -43.5869) knots 0 0 0 0 0.068378 0.147723 0.147723 0.147723 0.147723
  spline S58 degree 3 poles (2.5782, -43.5869) (2.2984, -43.5741) (1.779, -43.5504) (1.355, -43.2533) (1.1594, -43.1162) knots 0 0 0 0 0.082022 0.152248 0.152248 0.152248 0.152248
  spline S59 degree 3 poles (1.1594, -43.1162) (1.0122, -42.9448) (0.7106, -42.5937) (0.6736, -42.1317) (0.6546, -41.8952) knots 0 0 0 0 0.065997 0.135199 0.135199 0.135199 0.135199
  spline S60 degree 3 poles (0.6546, -41.8952) (0.6734, -41.6658) (0.7104, -41.2162) (1.0049, -40.8752) (1.1491, -40.7083) knots 0 0 0 0 0.067144 0.131583 0.131583 0.131583 0.131583
  spline S61 degree 3 poles (1.1491, -40.7083) (1.3409, -40.5742) (1.757, -40.2833) (2.2662, -40.2603) (2.5407, -40.2478) knots 0 0 0 0 0.068809 0.149275 0.149275 0.149275 0.149275
  spline S62 degree 3 poles (2.5407, -40.2478) (2.5634, -40.2481) (2.618, -40.2486) (2.6726, -40.2503) (2.7044, -40.2513) knots 0 0 0 0 0.006822 0.016375 0.016375 0.016375 0.016375
  line L65 (2.7044, -40.2513) -> (2.7044, -42.9525)
  spline S63 degree 3 poles (2.7044, -42.9525) (2.8862, -42.9347) (3.2218, -42.902) (3.4938, -42.705) (3.6184, -42.6148) knots 0 0 0 0 0.053662 0.09901 0.09901 0.09901 0.09901
  spline S64 degree 3 poles (3.6184, -42.6148) (3.7109, -42.5067) (3.8977, -42.2884) (3.9229, -42.0021) (3.9356, -41.8577) knots 0 0 0 0 0.041583 0.083942 0.083942 0.083942 0.083942
  line L66 (4.3585, -48.0241) -> (4.3585, -48.6653)
  spline S65 degree 3 poles (4.3585, -48.6653) (4.2903, -48.6945) (4.1471, -48.7557) (3.9926, -48.777) (3.9117, -48.7881) knots 0 0 0 0 0.022155 0.046521 0.046521 0.046521 0.046521
  spline S66 degree 3 poles (3.9117, -48.7881) (3.9995, -48.8963) (4.1634, -49.0983) (4.2711, -49.3349) (4.321, -49.4446) knots 0 0 0 0 0.041611 0.077646 0.077646 0.077646 0.077646
  spline S67 degree 3 poles (4.321, -49.4446) (4.3558, -49.5528) (4.4267, -49.7729) (4.4358, -50.004) (4.4404, -50.1217) knots 0 0 0 0 0.033903 0.069032 0.069032 0.069032 0.069032
  spline S68 degree 3 poles (4.4404, -50.1217) (4.4331, -50.3033) (4.4198, -50.6373) (4.2337, -50.9133) (4.1488, -51.0391) knots 0 0 0 0 0.053281 0.097966 0.097966 0.097966 0.097966
  spline S69 degree 3 poles (4.1488, -51.0391) (4.0439, -51.1326) (3.8313, -51.3221) (3.5474, -51.3471) (3.4036, -51.3597) knots 0 0 0 0 0.041002 0.083083 0.083083 0.083083 0.083083
  spline S70 degree 3 poles (3.4036, -51.3597) (3.3174, -51.355) (3.1476, -51.3457) (2.9934, -51.2739) (2.9175, -51.2386) knots 0 0 0 0 0.025631 0.050498 0.050498 0.050498 0.050498
  spline S71 degree 3 poles (2.9175, -51.2386) (2.8482, -51.1957) (2.7115, -51.111) (2.613, -50.984) (2.5645, -50.9214) knots 0 0 0 0 0.02426 0.047798 0.047798 0.047798 0.047798
  spline S72 degree 3 poles (2.5645, -50.9214) (2.5227, -50.8533) (2.4374, -50.7144) (2.3883, -50.5589) (2.3633, -50.4798) knots 0 0 0 0 0.023897 0.048698 0.048698 0.048698 0.048698
  spline S73 degree 3 poles (2.3633, -50.4798) (2.3467, -50.4043) (2.3069, -50.224) (2.2844, -50.0407) (2.2712, -49.9341) knots 0 0 0 0 0.023161 0.055369 0.055369 0.055369 0.055369
  spline S74 degree 3 poles (2.2712, -49.9341) (2.245, -49.7177) (2.2002, -49.3475) (2.101, -48.9884) (2.0598, -48.8393) knots 0 0 0 0 0.065274 0.111639 0.111639 0.111639 0.111639
  spline S75 degree 3 poles (2.0598, -48.8393) (2.0254, -48.8383) (1.972, -48.8368) (1.9185, -48.8361) (1.8995, -48.8358) knots 0 0 0 0 0.01032 0.016034 0.016034 0.016034 0.016034
  spline S76 degree 3 poles (1.8995, -48.8358) (1.7885, -48.8383) (1.5929, -48.8426) (1.4379, -48.9593) (1.3708, -49.0098) knots 0 0 0 0 0.032269 0.056898 0.056898 0.056898 0.056898
  spline S77 degree 3 poles (1.3708, -49.0098) (1.3103, -49.1046) (1.175, -49.3166) (1.1671, -49.5692) (1.1628, -49.709) knots 0 0 0 0 0.033148 0.074151 0.074151 0.074151 0.074151
  spline S78 degree 3 poles (1.1628, -49.709) (1.1648, -49.8372) (1.1683, -50.0626) (1.2705, -50.2624) (1.3145, -50.3485) knots 0 0 0 0 0.037836 0.066498 0.066498 0.066498 0.066498
  spline S79 degree 3 poles (1.3145, -50.3485) (1.3811, -50.4142) (1.532, -50.5632) (1.7371, -50.6213) (1.8517, -50.6537) knots 0 0 0 0 0.027639 0.062674 0.062674 0.062674 0.062674
  line L67 (1.8517, -50.6537) -> (1.7699, -51.254)
  spline S80 degree 3 poles (1.7699, -51.254) (1.6507, -51.2247) (1.4278, -51.1699) (1.2365, -51.0434) (1.1474, -50.9845) knots 0 0 0 0 0.036476 0.068275 0.068275 0.068275 0.068275
  spline S81 degree 3 poles (1.1474, -50.9845) (1.0719, -50.9119) (0.9114, -50.7577) (0.8271, -50.5514) (0.7825, -50.4423) knots 0 0 0 0 0.031081 0.066011 0.066011 0.066011 0.066011
  spline S82 degree 3 poles (0.7825, -50.4423) (0.7452, -50.3155) (0.6664, -50.0473) (0.6587, -49.7677) (0.6546, -49.6203) knots 0 0 0 0 0.039468 0.083496 0.083496 0.083496 0.083496
  spline S83 degree 3 poles (0.6546, -49.6203) (0.657, -49.4791) (0.6613, -49.2229) (0.732, -48.977) (0.7637, -48.8665) knots 0 0 0 0 0.042125 0.076454 0.076454 0.076454 0.076454
  spline S84 degree 3 poles (0.7637, -48.8665) (0.7993, -48.7791) (0.8643, -48.6194) (0.9841, -48.496) (1.0383, -48.4402) knots 0 0 0 0 0.028009 0.05113 0.05113 0.05113 0.05113
  spline S85 degree 3 poles (1.0383, -48.4402) (1.0989, -48.3978) (1.2263, -48.3085) (1.3771, -48.2696) (1.4561, -48.2492) knots 0 0 0 0 0.022017 0.046272 0.046272 0.046272 0.046272
  spline S86 degree 3 poles (1.4561, -48.2492) (1.5293, -48.2404) (1.7173, -48.2177) (1.9067, -48.2182) (2.0223, -48.2185) knots 0 0 0 0 0.022119 0.056745 0.056745 0.056745 0.056745
  line L68 (2.0223, -48.2185) -> (2.8408, -48.2185)
  spline S87 degree 3 poles (2.8408, -48.2185) (3.0739, -48.2199) (3.4356, -48.2221) (3.7957, -48.1905) (3.9237, -48.1793) knots 0 0 0 0 0.069882 0.108407 0.108407 0.108407 0.108407
  spline S88 degree 3 poles (3.9237, -48.1793) (3.9988, -48.1629) (4.1504, -48.1297) (4.2887, -48.0595) (4.3585, -48.0241) knots 0 0 0 0 0.022967 0.046339 0.046339 0.046339 0.046339
  line L69 (4, 28) -> (30.0228, 28)
  line L70 (30.0228, 28) -> (30.0228, 6.8336)
  line L71 (30.0228, 6.8336) -> (4, 6.8336)
  line L72 (4, 6.8336) -> (4, 28)
  arc A9 (-10.8289, -17.7317) -> (-11.3289, -17.2317) centre (-11.3289, -17.7317) ccw
  arc A10 (-9.3925, -18.5415) -> (-9.6425, -18.2915) centre (-9.6425, -18.5415) ccw
  line L73 (-6.6003, -20.9602) -> (-6.6003, -58.5213)
  arc A11 (-8.6003, -19.9602) -> (-9.3925, -20.3499) centre (-8.6003, -20.9602) ccw
  line L74 (-8.6003, -19.9602) -> (-7.6003, -19.9602)
  arc A12 (-6.6003, -20.9602) -> (-7.6003, -19.9602) centre (-7.6003, -20.9602) ccw
  constraint horizontal L69
  constraint vertical L70
  constraint horizontal L71
  constraint vertical L72
extrude "Extrude16" cut sketch "Sketch11" against normal blind 1.5 contours L69 L70 L71 L72 bodies 1
fillet "Fillet9" radius 4 1 edges at (-30.0228, -17.4168, 0) on bodies 1
sketch "Sketch12" plane through (0, 0, 20) normal (0, 0, 1) x (-1, 0, 0)
  line L0 (59, -69.6198) -> (60, -68.6198)
  line L1 (60, -68.6198) -> (60, -21.7915)
  line L2 (60, -21.7915) -> (59.9993, -21.7915)
  line L3 (59.9993, -21.7915) -> (59.9993, 34)
  line L4 (59.9993, 34) -> (58.9993, 35)
  line L5 (58.9993, 35) -> (-38, 35)
  line L6 (-38, 35) -> (-39, 34)
  line L7 (-39, 34) -> (-39, -68.6198)
  line L8 (-39, -68.6198) -> (-38, -69.6198)
  line L9 (-38, -69.6198) -> (-35.8045, -69.6198)
  line L10 (-35.8045, -69.6198) -> (-35.8045, -20.4602)
  line L11 (-35.8045, -20.4602) -> (-36.8615, -20.4602)
  line L12 (-36.8615, -20.4602) -> (-36.8615, -18.2915)
  line L13 (-36.8615, -18.2915) -> (-11.3289, -18.2915)
  arc A0 (-11.3289, -18.2915) -> (-10.8289, -17.7915) centre (-11.3289, -17.7915) ccw
  line L14 (-10.8289, -17.7915) -> (-10.8289, -17.7317)
  arc A1 (-10.8289, -17.7317) -> (-11.3289, -17.2317) centre (-11.3289, -17.7317) ccw
  line L15 (-11.3289, -17.2317) -> (-36.8727, -17.2317)
  line L16 (-36.8727, -17.2317) -> (-36.8727, 33)
  line L17 (-36.8727, 33) -> (2.3035, 33)
  line L18 (2.3035, 33) -> (2.3035, 34.4706)
  line L19 (2.3035, 34.4706) -> (21.6224, 34.4706)
  line L20 (21.6224, 34.4706) -> (21.6224, 33)
  line L21 (21.6224, 33) -> (57.9993, 33)
  line L22 (57.9993, 33) -> (57.9993, -17.2317)
  line L23 (57.9993, -17.2317) -> (32.3289, -17.2317)
  arc A2 (32.3289, -17.2317) -> (31.8289, -17.7317) centre (32.3289, -17.7317) ccw
  line L24 (31.8289, -17.7317) -> (31.8289, -17.7915)
  arc A3 (31.8289, -17.7915) -> (32.3289, -18.2915) centre (32.3289, -17.7915) ccw
  line L25 (32.3289, -18.2915) -> (57.8615, -18.2915)
  line L26 (57.8615, -18.2915) -> (57.8615, -20.4602)
  line L27 (57.8615, -20.4602) -> (56.8045, -20.4602)
  line L28 (56.8045, -20.4602) -> (56.8045, -69.6198)
  line L29 (56.8045, -69.6198) -> (59, -69.6198)
  line L30 (-38, 35) -> (58.9993, 35)
  line L31 (60, -21.7915) -> (60, -68.6198)
  line L32 (59, -69.6198) -> (-38, -69.6198)
  line L33 (-39, -68.6198) -> (-39, 34)
  line L34 (59, -69.6198) -> (60, -68.6198)
  line L35 (-39, -68.6198) -> (-38, -69.6198)
  line L36 (-39, 34) -> (-38, 35)
  line L37 (58.9993, 35) -> (59.9993, 34)
  circle A4 centre (22.1013, -52.8172) radius 2.0273
  circle A5 centre (22.1, -27.4) radius 2.0133
  constraint horizontal L30
  constraint vertical L31
  constraint horizontal L32
  constraint vertical L33
  constraint coincident L0.start L29.end
  constraint coincident L0.end L1.start
  constraint coincident L7.end L8.start
  constraint coincident L8.end L9.start
  constraint coincident L6.end L7.start
  constraint coincident L5.end L6.start
  constraint coincident L4.end L5.start
  constraint coincident L3.end L4.start
extrude "Extrude17" add sketch "Sketch12" along normal blind 2 separate body makes body 2
move_body "Move1" bodies 2 to x (1, 0, 0) y (0, 1, 0) z (0, 0, 1) at (115, 0, 0)
sketch "Sketch13" plane through (0, 0, -4) normal (0, 0, -1) x (1, 0, 0)
  line L0 (-59, 35) -> (-60, 34)
  line L1 (-60, 34) -> (-60, -68.6198)
  line L2 (-60, -68.6198) -> (-59, -69.6198)
  line L3 (-59, -69.6198) -> (38, -69.6198)
  line L4 (38, -69.6198) -> (39, -68.6198)
  line L5 (39, -68.6198) -> (39, 34)
  line L6 (39, 34) -> (38, 35)
  line L7 (38, 35) -> (-59, 35)
  line L8 (-57.1659, -20.3442) -> (36.7375, -20.1545) construction
  line L9 (36.7375, -20.1545) -> (36.6365, 29.8312) construction
  line L10 (36.6365, 29.8312) -> (-57.2668, 29.6415) construction
  line L11 (-57.2668, 29.6415) -> (-57.1659, -20.3442) construction
  line L12 (10, -67.8581) -> (35.2612, -67.8581) construction
  line L13 (35.2612, -67.8581) -> (35.2612, -55) construction
  line L14 (35.2612, -55) -> (10, -55) construction
  line L15 (10, -55) -> (10, -67.8581) construction
  line L16 (-55, -67.8581) -> (-29.7388, -67.8581) construction
  line L17 (-29.7388, -67.8581) -> (-29.7388, -55) construction
  line L18 (-29.7388, -55) -> (-55, -55) construction
  line L19 (-55, -55) -> (-55, -67.8581) construction
  dimension "d102" = 9.5
  dimension "d104" = 5.5
  dimension "d106" = 5.5
  text T0 "NeoLabs\nLaunch System\nV2" font "Arial" height 9.5 align centre middle in box 93.9035 x 49.9858 at (-57.1659, -20.3442) x (0.999998, 0.00202) y (-0.00202, 0.999998) spacing 1 kerned
  text T1 "PWR" font "Arial" height 5.5 align centre middle in box 25.2612 x 12.8581 at (10, -67.8581) x (1, 0) y (0, 1) spacing 1 kerned
  text T2 "GLOW" font "Arial" height 5.5 align centre middle in box 25.2612 x 12.8581 at (-55, -67.8581) x (1, 0) y (0, 1) spacing 1 kerned
extrude "Extrude18" cut sketch "Sketch13" against normal blind 0.5 text T2 T1 T0 bodies 1
equation "d1 = 65 mm + 32 mm + 2 mm"
equation "d89 = 'Made by Neo'"
equation "d103 = 'NeoLabs Launch System V2'"
equation "d105 = 'PWR'"
equation "d107 = 'GLOW'"
